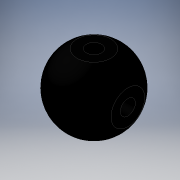
# Autodesk Inventor part: xyz_Axis_with_ball_Ball
Saved by Autodesk Inventor 2018.2 (Build 222227000, 227)
## iProperties
Created: 2018-06-07
Part Number: xyz_Axis_with_ball_Ball
Material: Generisch
Document SubType Name: Modeling
Designer: Nick Koch
Density: 1 g/cm^3
Appearance: Vorgabe
Author: Nick Koch
Autodesk Inventor part; units mm, degrees
ref_plane "YZ Plane" through (0, 0, 0) normal (1, 0, 0) x (0, 1, 0)
sketch "Skizze1" plane through (0, 0, 0) normal (0, 0, 1) x (1, 0, 0)
  circle A0 centre (0, 0) radius 2.5
  line L0 (0, 2.5) -> (0, -2.5)
  dimension "d0" = 5
  constraints: 2 end point, 2 point on circle, 1 centre point, 1 coincident, 1 vertical
  measures "d0" diameter of A0
revolve "Umdrehung1" add sketch "Skizze1" angle 360 about axis through (0, 2.5, 0) along (0, -1, 0) picked at (0.5196, 0.6515) contours A0 L0
ref_plane "Arbeitsebene1" through (0, 0, 0) normal (-1, 0, 0) x (0, -1, 0)
sketch "Skizze2" plane through (0, 0, 0) normal (-1, 0, 0) x (0, -1, 0)
  circle A0 centre (0, 0) radius 2.5 projected
  line L0 (1.8885, 2.6999) -> (-1.1115, 2.6999)
  line L1 (-1.1115, 2.6999) -> (-1.1115, 2.2393)
  line L2 (-1.1115, 2.2393) -> (1.8885, 2.2393)
  line L3 (1.8885, 2.2393) -> (1.8885, 2.6999)
  line L4 (1.8885, 2.6999) -> (-1.1115, 2.2393) construction
  line L5 (-1.1115, 2.6999) -> (1.8885, 2.2393) construction
  point P0 (0.3885, 2.4696)
  dimension "d2" = 3
  constraints: 12 end point, 2 midpoint, 2 parallel, 2 point on circle, 1 horizontal, 1 perpendicular
  measures "d2" distance of L2.end L1.end
extrude "Extrusion1" cut sketch "Skizze2" along normal mid plane 10 contours L1 L0 L3 L2 A0 | A0 L2 picked at (0.1903, 2.3042)
ref_plane "Arbeitsebene2" through (0, 0, 2.2393) normal (0, -1, 0) x (-1, 0, 0)
sketch "Skizze3" plane through (0, 0, 2.2393) normal (0, -1, 0) x (-1, 0, 0)
  arc A0 (1.1115, 0) -> (-1.1115, 0) centre (0, 2.2393) ccw projected
  line L0 (-2.6999, 0.3508) -> (-2.2393, 0.3508)
  line L1 (-2.2393, 0.3508) -> (-2.2393, 3.3508)
  line L2 (-2.2393, 3.3508) -> (-2.6999, 3.3508)
  line L3 (-2.6999, 3.3508) -> (-2.6999, 0.3508)
  line L4 (-2.6999, 0.3508) -> (-2.2393, 3.3508) construction
  line L5 (-2.2393, 0.3508) -> (-2.6999, 3.3508) construction
  point P0 (-2.4696, 1.8508)
  dimension "d5" = 3
  constraints: 12 end point, 2 midpoint, 2 parallel, 2 point on circle, 1 horizontal, 1 perpendicular
  measures "d5" distance of L1.end L0.end
extrude "Extrusion2" cut sketch "Skizze3" along normal mid plane 10
sketch "Skizze4" plane through (0, 0, 0) normal (-1, 0, 0) x (0, -1, 0)
  arc A0 (-1.1115, 2.2393) -> (1.1115, 2.2393) centre (0, 0) ccw projected
  line L0 (-2.6999, 1.8885) -> (-2.2393, 1.8885)
  line L1 (-2.2393, 1.8885) -> (-2.2393, -1.1115)
  line L2 (-2.2393, -1.1115) -> (-2.6999, -1.1115)
  line L3 (-2.6999, -1.1115) -> (-2.6999, 1.8885)
  line L4 (-2.6999, 1.8885) -> (-2.2393, -1.1115) construction
  line L5 (-2.2393, 1.8885) -> (-2.6999, -1.1115) construction
  point P0 (-2.4696, 0.3885)
  dimension "d8" = 3
  constraints: 12 end point, 2 midpoint, 2 parallel, 2 point on circle, 1 horizontal, 1 perpendicular
  measures "d8" distance of L0.end L1.end
extrude "Extrusion3" cut sketch "Skizze4" along normal mid plane 10
sketch "Skizze5" plane through (2.2393, 0, 0) normal (1, 0, 0) x (0, 0, -1)
  circle A0 centre (0, 0) radius 1.1115
  circle A1 centre (0, 0) radius 0.5
  dimension "d26" = 1
  constraints: 2 centre point, 2 coincident
  measures "d26" diameter of A1
sketch "Skizze6" plane through (0, 0, 2.2393) normal (0, 0, 1) x (1, 0, 0)
  circle A0 centre (0, 0) radius 1.1115
  circle A1 centre (0, 0) radius 0.5
  dimension "d27" = 1
  constraints: 2 centre point, 2 coincident
  measures "d27" diameter of A1
sketch "Skizze7" plane through (0, 2.2393, 0) normal (0, 1, 0) x (1, 0, 0)
  circle A0 centre (0, 0) radius 1.1115
  circle A1 centre (0, 0) radius 0.5
  dimension "d28" = 1
  constraints: 2 centre point, 2 coincident
  measures "d28" diameter of A1
extrude "Extrusion7" cut sketch "Skizze6" against normal blind 1.5 contours A1
extrude "Extrusion8" cut sketch "Skizze5" against normal blind 1.5 contours A1
extrude "Extrusion9" cut sketch "Skizze7" against normal blind 1.5 contours A1
